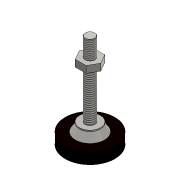
# Autodesk Inventor part: Adjuster Pad
Saved by Autodesk Inventor 2016 (Build 200138000, 138)
## iProperties
Created: 2021-03-12
Part Number: Adjuster Pad
Material: Stainless Steel
Document SubType Name: Modeling
Designer: DRAFT 2
Density: 8 g/cm^3
Appearance: Semi-Polished
Author: DRAFT 2
Autodesk Inventor part; units mm, degrees
ref_plane "YZ Plane" through (0, 0, 0) normal (1, 0, 0) x (0, 1, 0)
ref_plane "XZ Plane" through (0, 0, 0) normal (0, 1, 0) x (-1, 0, 0)
ref_plane "XY Plane" through (0, 0, 0) normal (0, 0, 1) x (1, 0, 0)
sketch "Sketch1" plane through (0, 0, 0) normal (0, 0, 1) x (1, 0, 0)
  circle A0 centre (0, 0) radius 4
  dimension "d0" = 8
  constraints: 1 centre point, 1 coincident
  measures "d0" diameter of A0
extrude "Extrusion1" add sketch "Sketch1" along normal blind 54
sketch "Sketch2" plane through (0, 0, 0) normal (0, 0, -1) x (-1, 0, 0)
  line L0 (0, 7.5056) -> (6.5, 3.7528)
  line L1 (6.5, 3.7528) -> (6.5, -3.7528)
  line L2 (6.5, -3.7528) -> (0, -7.5056)
  line L3 (0, -7.5056) -> (-6.5, -3.7528)
  line L4 (-6.5, -3.7528) -> (-6.5, 3.7528)
  line L5 (-6.5, 3.7528) -> (0, 7.5056)
  point P0 (0, 0)
  point P1 (0, 0)
  dimension "d3" = 13
  dimension "d4" = 6.5
  constraints: 12 end point, 1 coincident, 13 other
  measures "d3" distance between parallel lines of L0 L3
  measures "d4" horizontal distance of L2.end L3.end
extrude "Extrusion2" add sketch "Sketch2" along normal blind 6
sketch "Sketch3" plane through (0, 0, -6) normal (0, 0, -1) x (-1, 0, 0)
  circle A0 centre (0, 0) radius 8.5
  dimension "d7" = 17
  constraints: 1 centre point, 1 coincident
  measures "d7" diameter of A0
extrude "Extrusion3" add sketch "Sketch3" along normal blind 1
sketch "Sketch4" plane through (0, 0, -7) normal (0, 0, -1) x (-1, 0, 0)
  circle A0 centre (0, 0) radius 7.5
  dimension "d10" = 15
  constraints: 1 centre point, 1 coincident
  measures "d10" diameter of A0
ref_plane "Work Plane1" through (0, 0, -17) normal (0, 0, -1) x (-1, 0, 0)
sketch "Sketch5" plane through (0, 0, -17) normal (0, 0, -1) x (-1, 0, 0)
  circle A0 centre (0, 0) radius 14.5
  dimension "d12" = 29
  constraints: 1 centre point, 1 coincident
  measures "d12" diameter of A0
loft "Loft1" add profiles "Sketch4", "Sketch5"
sketch "Sketch6" plane through (0, 0, -17) normal (0, 0, -1) x (-1, 0, 0)
  circle A0 centre (0, 0) radius 17
  dimension "d17" = 34
  constraints: 1 centre point, 1 coincident
  measures "d17" diameter of A0
extrude "Extrusion4" add sketch "Sketch6" against normal blind 2
chamfer "Chamfer1" distance 0.3 angle 45 1 edges at (-4, 0, 54)
sketch "Sketch7" plane through (0, 0, -17) normal (0, 0, -1) x (-1, 0, 0)
  circle A0 centre (0, 0) radius 4 projected
  circle A1 centre (0, 0) radius 20
  dimension "d26" = 40
  constraints: 1 centre point, 1 coincident
  measures "d26" diameter of A1
extrude "Extrusion5" add sketch "Sketch7" against normal blind 4 and the other way blind 5
sketch "Sketch8" plane through (0, 0, -22) normal (0, 0, -1) x (-1, 0, 0)
  circle A0 centre (0, 0) radius 8
  dimension "d31" = 16
  constraints: 1 centre point, 1 coincident
  measures "d31" diameter of A0
extrude "Extrusion6" cut sketch "Sketch8" against normal blind 12
sketch "Sketch9" plane through (0, 0, 0) normal (0, 0, 1) x (1, 0, 0)
  line L0 (0, 7.5056) -> (-6.5, 3.7528) projected
  line L1 (-6.5, 3.7528) -> (-6.5, -3.7528) projected
  line L2 (-6.5, -3.7528) -> (0, -7.5056) projected
  line L3 (0, -7.5056) -> (6.5, -3.7528) projected
  line L4 (6.5, -3.7528) -> (6.5, 3.7528) projected
  line L5 (6.5, 3.7528) -> (0, 7.5056) projected
  circle A0 centre (0, 0) radius 4 projected
extrude "Extrusion7" cut sketch "Sketch9" against normal up to surface (6 mm away)
ref_plane "Work Plane2" through (0, 0, 39) normal (0, 0, 1) x (1, 0, 0)
sketch "Sketch10" plane through (0, 0, 39) normal (0, 0, 1) x (1, 0, 0)
  circle A0 centre (0, 0) radius 4 projected
  line L0 (8.6603, 0) -> (4.3301, -7.5)
  line L1 (4.3301, -7.5) -> (-4.3301, -7.5)
  line L2 (-4.3301, -7.5) -> (-8.6603, 0)
  line L3 (-8.6603, 0) -> (-4.3301, 7.5)
  line L4 (-4.3301, 7.5) -> (4.3301, 7.5)
  line L5 (4.3301, 7.5) -> (8.6603, 0)
  dimension "d37" = 15
  dimension "d38" = 8.6602
  dimension "d39" = 8.6602
  constraints: 12 end point, 1 coincident, 13 other
  measures "d37" distance between parallel lines of L1 L4
  measures "d38" distance of L4.end L0.start
  measures "d39" distance of L3.end L4.end
extrude "Extrusion8" add sketch "Sketch10" against normal blind 5.5
thread "Thread2" size "M8x1.25" class "6g" standard "ISO Metric profile" full length
thread "Thread3" size "M10x1.5" class "6g" standard "ANSI Metric M Profile" full length
equation "\"d4\" = 0.5 * d3"
body "Solid1"
